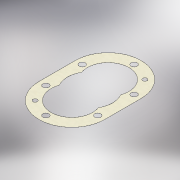
# Autodesk Inventor part: 垫片
Saved by Autodesk Inventor 2020 (Build 240168000, 168)
## iProperties
Created: 2021-04-21
Part Number: 垫片
Material: 纸
Document SubType Name: Modeling
Designer: Luorily
Density: 0.93 g/cm^3
Appearance: 卡纸板 - 刨花板
Author: Luorily
Autodesk Inventor part; units mm, degrees
ref_plane "YZ Plane" through (0, 0, 0) normal (1, 0, 0) x (0, 1, 0)
ref_plane "XZ Plane" through (0, 0, 0) normal (0, 1, 0) x (-1, 0, 0)
ref_plane "XY Plane" through (0, 0, 0) normal (0, 0, 1) x (1, 0, 0)
sketch "草图1" plane through (0, 0, 0) normal (0, 1, 0) x (-1, 0, 0)
  line L0 (38, 21) -> (38, -21)
  line L1 (-38, 21) -> (-38, -21)
  circle A0 centre (0, 51) radius 3.5
  circle A1 centre (30, 21) radius 3.5
  circle A2 centre (-30, 21) radius 3.5
  circle A3 centre (-30, -21) radius 3.5
  circle A4 centre (0, -51) radius 3.5
  circle A5 centre (30, -21) radius 3.5
  line L2 (0, 21) -> (30, 21) construction
  line L3 (0, -21) -> (-21.2132, -42.2132)
  line L4 (0, -21) -> (30, -21) construction
  circle A6 centre (21.2132, 42.2132) radius 2.5
  circle A7 centre (-21.2132, -42.2132) radius 2.5
  arc A8 (22.585, -12.881) -> (22.585, 12.881) centre (0, 0) ccw
  arc A9 (-22.585, 12.881) -> (-22.585, -12.881) centre (0, 0) ccw
  line L5 (16.9706, 37.9706) -> (21.2132, 42.2132)
  line L6 (0, 21) -> (0, 17)
  line L7 (0, 3) -> (0, -21)
  line L8 (0, 0) -> (0, 3)
  line L9 (0, 17) -> (0, 21)
  arc A10 (-22.585, -12.881) -> (22.585, -12.881) centre (0, -21) ccw
  arc A11 (16.7965, -3.8571) -> (11.619, 0) centre (0, -21) ccw
  arc A12 (-29.7958, -17.506) -> (29.7958, -17.506) centre (0, -21) ccw
  arc A13 (21.4243, 0) -> (16.7965, 3.8571) centre (0, -21) ccw
  arc A14 (16.7965, -3.8571) -> (21.4243, 0) centre (0, 21) ccw
  arc A15 (11.619, 0) -> (16.7965, 3.8571) centre (0, 21) ccw
  arc A16 (22.585, 12.881) -> (-22.585, 12.881) centre (0, 21) ccw
  arc A17 (38, 21) -> (-38, 21) centre (0, 21) ccw
  arc A18 (-24.8069, 7.7857) -> (-26.2499, 6.4762) centre (0, -21) ccw
  arc A19 (-38, -21) -> (38, -21) centre (0, -21) ccw
  arc A20 (29.7958, 17.506) -> (-29.7958, 17.506) centre (0, 21) ccw
  arc A21 (-26.2499, 6.4762) -> (-25.4815, 5.1667) centre (0, 21) ccw
  dimension "d8" = 7
  dimension "d9" = 7
  dimension "d10" = 7
  dimension "d13" = 7
  dimension "d0" = 21
  dimension "d1" = 42
  dimension "d7" = 7
  dimension "d11" = 7
  dimension "d15" = 135
  dimension "d16" = 5
  dimension "d17" = 5
  constraints: 39 point on circle, 20 end point, 18 centre point, 8 coincident, 3 vertical, 2 horizontal, 2 tangent, 1 equal length, 1 parallel, 12 other
  measures "d0" distance of L8.start L6.start
  measures "d1" distance of L6.start L7.end
  measures "d7" diameter of A0
  measures "d11" diameter of A4
  measures "d15" angle of L3 L4
  measures "d16" diameter of A6
  measures "d17" diameter of A7
extrude "拉伸1" add sketch "草图1" along normal blind 0.05 contours L0 A19 L1 A17 | A9 A21 A18
